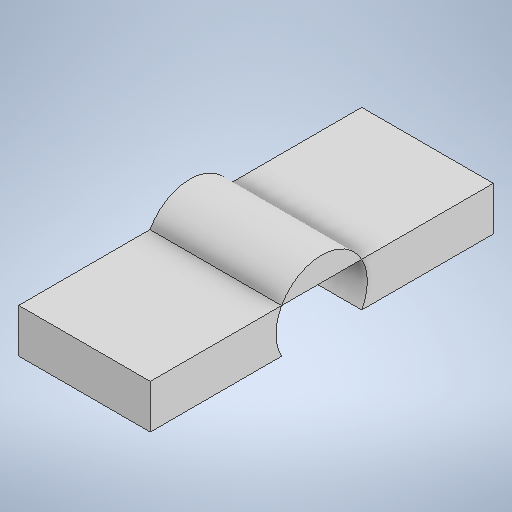
# Autodesk Inventor part: secures
Saved by Autodesk Inventor 2025.3 (Build 293356030, 356C)
## iProperties
Created: 2026-06-24
Part Number: secures
Material: Generic
Document SubType Name: Modeling
Designer: user
Density: 1 g/cm^3
Appearance: Default
Author: user
Autodesk Inventor part; units mm, degrees
ref_plane "YZ Plane" through (0, 0, 0) normal (1, 0, 0) x (0, 1, 0)
ref_plane "XZ Plane" through (0, 0, 0) normal (0, 1, 0) x (-1, 0, 0)
ref_plane "XY Plane" through (0, 0, 0) normal (0, 0, 1) x (1, 0, 0)
sketch "Sketch1" plane through (0, 0, 0) normal (1, 0, 0) x (0, 1, 0)
  line L0 (0, 0) -> (10, 0)
  line L1 (10, 0) -> (10, -30)
  line L2 (0, 0) -> (0, -20)
  arc A0 (0, -48.1907) -> (0, -29.9291) centre (5, -39.0599) ccw
  line L3 (10, -48.1907) -> (10, -78.1907)
  line L4 (10, -78.1907) -> (0, -78.1907)
  line L5 (0, -78.1907) -> (0, -48.1907)
  line L6 (0, -29.9291) -> (0, -20)
  line L7 (10, -48.1907) -> (10, -30)
  point P0 (10, -29.9291)
  dimension "d0" = 10
  dimension "d1" = 30
  dimension "d2" = 20
  dimension "d3" = 30
  constraints: 16 end point, 4 point on circle, 3 vertical, 2 perpendicular, 1 centre point, 1 collinear, 1 horizontal, 1 point on line
  measures "d0" distance of L0.start L0.end
  measures "d1" distance of L0.end L1.end
  measures "d2" distance of L0.start L2.end
  measures "d3" distance of L3.start L3.end
extrude "Extrusion1" add sketch "Sketch1" along normal blind 30
body "Solid1"
